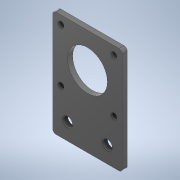
# Autodesk Inventor part: pad dong co buoc truc Y
Saved by Autodesk Inventor 2020 (Build 240168000, 168)
## iProperties
Created: 2021-05-28
Part Number: pad dong co buoc truc Y
Material: Generic
Document SubType Name: Modeling
Designer: admin
Density: 1 g/cm^3
Appearance: Smooth - Black
Author: admin
Autodesk Inventor part; units mm, degrees
ref_plane "YZ Plane" through (0, 0, 0) normal (1, 0, 0) x (0, 1, 0)
ref_plane "XZ Plane" through (0, 0, 0) normal (0, 1, 0) x (-1, 0, 0)
ref_plane "XY Plane" through (0, 0, 0) normal (0, 0, 1) x (1, 0, 0)
sketch "Sketch1" plane through (0, 0, 0) normal (0, 0, 1) x (1, 0, 0)
  line L0 (-21, -32) -> (21, -32)
  line L1 (21, -32) -> (21, 32)
  line L2 (21, 32) -> (-21, 32)
  line L3 (-21, 32) -> (-21, -32)
  line L4 (-21, -32) -> (21, 32) construction
  line L5 (21, -32) -> (-21, 32) construction
  circle A0 centre (0, 11) radius 12
  circle A1 centre (-12, -22) radius 3
  circle A2 centre (12, -22) radius 3
  line L6 (-16, -5) -> (16, -5)
  line L7 (16, -5) -> (16, 27)
  line L8 (16, 27) -> (-16, 27)
  line L9 (-16, 27) -> (-16, -5)
  line L10 (-16, -5) -> (16, 27) construction
  line L11 (16, -5) -> (-16, 27) construction
  circle A3 centre (-16, 27) radius 1.75
  circle A4 centre (16, 27) radius 1.75
  circle A5 centre (16, -5) radius 1.75
  circle A6 centre (-16, -5) radius 1.75
  point P0 (0, 0)
  dimension "d0" = 42
  dimension "d1" = 64
  dimension "d2" = 43
  dimension "d3" = 21
  dimension "d4" = 24
  dimension "d5" = 6
  dimension "d6" = 6
  dimension "d7" = 10
  dimension "d8" = 10
  dimension "d9" = 12
  dimension "d10" = 12
  dimension "d11" = 32
  dimension "d12" = 32
  dimension "d13" = 3.5
  dimension "d14" = 3.5
  dimension "d15" = 3.5
  dimension "d16" = 3.5
  constraints: 24 end point, 7 centre point, 4 coincident, 4 midpoint, 4 parallel, 2 horizontal, 2 perpendicular
  measures "d0" distance of L2.end L1.end
  measures "d1" distance of L1.end L0.end
  measures "d2" distance from line of L0 A0.centre
  measures "d3" distance from line of L1 A0.centre
  measures "d4" diameter of A0
  measures "d5" diameter of A1
  measures "d6" diameter of A2
  measures "d7" distance from line of L0 A1.centre
  measures "d8" distance from line of L0 A2.centre
  measures "d9" horizontal distance of A1.centre point (0, 0)
  measures "d10" horizontal distance of point (0, 0) A2.centre
  measures "d11" distance of L8.end L7.end
  measures "d12" distance of L7.end L6.end
  measures "d13" diameter of A3
  measures "d14" diameter of A4
  measures "d15" diameter of A5
  measures "d16" diameter of A6
extrude "Extrusion1" add sketch "Sketch1" along normal blind 3 contours L3 L2 L1 L0 | A6 L9 A3 L8 A4 L7 A5 L6
fillet "Fillet1" radius 2 4 edges at (-21, 32, 1.5) (21, 32, 1.5) (21, -32, 1.5) (-21, -32, 1.5)
body "Solid1"
